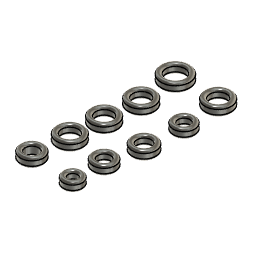
Ring Test v2 (Autodesk Fusion 360 design; units mm, degrees)
Autodesk Fusion 360 part; units mm, degrees
sketch "Skizze1" plane through (0, 0, 0) normal (0, 0, 1) x (1, 0, 0)
  circle A0 centre (-55, 0) radius 8.75
  circle A1 centre (-55, 0) radius 13.75
  circle A2 centre (-10, 0) radius 6.25
  circle A3 centre (-10, 0) radius 11.25
  circle A4 centre (-59, 40) radius 10
  circle A5 centre (-59, 40) radius 15
  circle A6 centre (-14, 40) radius 8.75
  circle A7 centre (-14, 40) radius 13.75
  circle A8 centre (-58, -36) radius 8.75
  circle A9 centre (-58, -36) radius 13.75
  circle A10 centre (-12, -40) radius 7.5
  circle A11 centre (-12, -40) radius 12.5
  circle A12 centre (-60, -70) radius 8.75
  circle A13 centre (-60, -70) radius 13.75
  circle A14 centre (-19, -75) radius 6.75
  circle A15 centre (-19, -75) radius 11.75
  circle A16 centre (-64, -106) radius 7
  circle A17 centre (-64, -106) radius 12
  circle A18 centre (-19, -108) radius 5
  circle A19 centre (-19, -108) radius 10
  dimension "d2" = 12.5
  dimension "d15" = 17.5
  dimension "d18" = 5
  dimension "d19" = 5
  dimension "d20" = 20
  dimension "d22" = 5
  dimension "d23" = 17.5
  dimension "d24" = 5
  dimension "d25" = 17.5
  dimension "d26" = 5
  dimension "d27" = 15
  dimension "d29" = 5
  dimension "d30" = 17.5
  dimension "d32" = 5
  dimension "d33" = 13.5
  dimension "d35" = 5
  dimension "d36" = 14
  dimension "d38" = 5
  dimension "d39" = 10
  dimension "d41" = 5
  constraint concentric A0 A1
  constraint concentric A2 A3
  constraint concentric A4 A5
  constraint concentric A6 A7
  constraint concentric A8 A9
  constraint concentric A10 A11
  constraint concentric A12 A13
  constraint concentric A14 A15
  constraint concentric A16 A17
  constraint concentric A18 A19
  measures "d2" diameter of A2
  measures "d15" diameter of A0
  measures "d18" distance of A0 A1
  measures "d19" distance of A2 A3
  measures "d20" diameter of A4
  measures "d22" distance of A4 A5
  measures "d23" diameter of A6
  measures "d24" distance of A6 A7
  measures "d25" diameter of A8
  measures "d26" distance of A8 A9
  measures "d27" diameter of A10
  measures "d29" distance of A10 A11
  measures "d30" diameter of A12
  measures "d32" distance of A12 A13
  measures "d33" diameter of A14
  measures "d35" distance of A14 A15
  measures "d36" diameter of A16
  measures "d38" distance of A16 A17
  measures "d39" diameter of A18
  measures "d41" distance of A18 A19
extrude "Extrusion2" add sketch "Skizze1" along normal blind 10 contours A5 | A7 makes body 1 at (-44.0186, 39.2523, 6.6667) makes body 2 at (-0.2671, 39.3146, 6.6667)
extrude "Extrusion3" add sketch "Skizze1" along normal blind 10 separate body contours A1 | A3 makes body 3 at (-41.2671, -0.6854, 6.6667) makes body 4 at (1.236, -0.5608, 6.6667)
extrude "Extrusion4" add sketch "Skizze1" along normal blind 10 separate body contours A9 | A11 makes body 5 at (-44.2671, -36.6854, 6.6667) makes body 6 at (0.4845, -40.6231, 6.6667)
extrude "Extrusion5" add sketch "Skizze1" along normal blind 10 separate body contours A13 | A15 makes body 7 at (-46.2671, -70.6854, 6.6667) makes body 8 at (-7.2646, -75.5857, 6.6667)
extrude "Extrusion6" add sketch "Skizze1" along normal blind 10 separate body contours A17 | A19 makes body 9 at (-52.0149, -106.5982, 6.6667) makes body 10 at (-9.0124, -108.4985, 6.6667)
fillet "Abrundung5" radius 2.5 20 edges at (-68.3233, 43.6162, 10) (-72.9849, 34.5758, 10) (-26.8195, 35.0278, 10) (-22.1579, 43.1641, 10) (-63.1579, 3.1641, 10) (-67.8195, -4.9722, 10) (-20.4887, -4.0682, 10) (-15.827, 2.2601, 10) (-70.8195, -40.9722, 10) (-66.1579, -32.8359, 10) (-18.9925, -37.2879, 10) (-23.6541, -44.5202, 10) (-68.1579, -66.8359, 10) (-72.8195, -74.9722, 10) (-29.9548, -79.249, 10) (-25.2932, -72.5591, 10) (-70.5263, -103.4687, 10) (-75.1879, -110.3394, 10) (-28.3233, -111.6162, 10) (-23.6616, -106.1919, 10) on bodies 1 2 3 4 5 6 7 8 9 10
fillet "Abrundung6" radius 2.5 19 edges at (-68.3233, 43.6162, 0) (-72.9849, 34.5758, 0) (-26.8195, 35.0278, 0) (-22.1579, 43.1641, 0) (-63.1579, 3.1641, 0) (-67.8195, -4.9722, 0) (-15.827, 2.2601, 0) (-20.4887, -4.0682, 0) (-66.1579, -32.8359, 0) (-70.8195, -40.9722, 0) (-23.6541, -44.5202, 0) (-18.9925, -37.2879, 0) (-68.1579, -66.8359, 0) (-72.8195, -74.9722, 0) (-29.9548, -79.249, 0) (-25.2932, -72.5591, 0) (-75.1879, -110.3394, 0) (-28.3233, -111.6162, 0) (-23.6616, -106.1919, 0) on bodies 1 2 3 4 5 6 7 8 9 10
equation "d2 = 15 mm - 2.5 mm"
named bodies: "Daumen_1", "Daume_2", "Zeigefinger_1", "Zeigefinger_2", "Mitelfinger_1", "Mitelfinger_2", "Ringfinger_1", "Ringinger_2", "Kleinerfinger_1", "Kleinerfinger_2"
